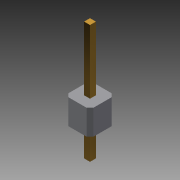
# Autodesk Inventor part: Pin
Saved by Autodesk Inventor 2013 SP1 (Build 170176100, 176)
## iProperties
Created: 2012-12-09
Part Number: Pin
Material: Allgemein
Document SubType Name: Modeling
Designer: Sebastian
Density: 1 g/cm^3
Author: Sebastian
Autodesk Inventor part; units mm, degrees
ref_plane "YZ Plane" through (0, 0, 0) normal (1, 0, 0) x (0, 1, 0)
ref_plane "XZ Plane" through (0, 0, 0) normal (0, 1, 0) x (-1, 0, 0)
ref_plane "XY Plane" through (0, 0, 0) normal (0, 0, 1) x (1, 0, 0)
sketch "Skizze1" plane through (0, 0, 0) normal (0, 0, 1) x (1, 0, 0)
  line L0 (-1.27, -1.27) -> (1.27, -1.27)
  line L1 (1.27, -1.27) -> (1.27, 1.27)
  line L2 (1.27, 1.27) -> (-1.27, 1.27)
  line L3 (-1.27, 1.27) -> (-1.27, -1.27)
  line L4 (-1.27, -1.27) -> (1.27, 1.27) construction
  line L5 (1.27, -1.27) -> (-1.27, 1.27) construction
  point P0 (0, 0)
  dimension "d0" = 2.54
  dimension "d1" = 2.54
  constraints: 12 end point, 2 midpoint, 2 parallel, 1 horizontal, 1 perpendicular
  measures "d0" distance of L2.end L1.end
  measures "d1" distance of L1.end L0.end
extrude "Extrusion1" add sketch "Skizze1" along normal blind 2.54
chamfer "Fase1" distance 0.35 angle 45 4 edges at (1.27, -1.27, 1.27) (-1.27, -1.27, 1.27) (-1.27, 1.27, 1.27) (1.27, 1.27, 1.27)
sketch "Skizze2" plane through (0, 0, 0) normal (0, 0, 1) x (1, 0, 0)
  line L0 (-0.3, -0.3) -> (0.3, -0.3)
  line L1 (0.3, -0.3) -> (0.3, 0.3)
  line L2 (0.3, 0.3) -> (-0.3, 0.3)
  line L3 (-0.3, 0.3) -> (-0.3, -0.3)
  line L4 (-0.3, -0.3) -> (0.3, 0.3) construction
  line L5 (0.3, -0.3) -> (-0.3, 0.3) construction
  point P0 (0, 0)
  dimension "d7" = 0.6
  dimension "d8" = 0.6
  constraints: 12 end point, 2 midpoint, 2 parallel, 1 horizontal, 1 perpendicular
  measures "d7" distance of L2.end L1.end
  measures "d8" distance of L1.end L0.end
extrude "Extrusion2" add sketch "Skizze2" along normal blind 9 and the other way blind 3 separate body
